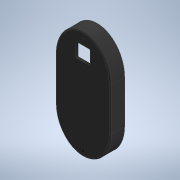
# Autodesk Inventor part: SpectoBoardCap
Saved by Autodesk Inventor 2020 (Build 240168000, 168)
## iProperties
Created: 2019-09-09
Part Number: SpectoBoardCap
Material: ABS Plastic
Document SubType Name: Modeling
Designer: vmiguel
Density: 1.06 g/cm^3
Appearance: Rubber - Black
Author: vmiguel
Autodesk Inventor part; units mm, degrees
ref_plane "YZ Plane" through (0, 0, 0) normal (1, 0, 0) x (0, 1, 0)
ref_plane "XZ Plane" through (0, 0, 0) normal (0, 1, 0) x (-1, 0, 0)
ref_plane "XY Plane" through (0, 0, 0) normal (0, 0, 1) x (1, 0, 0)
sketch "Sketch1" plane through (0, 0, 0) normal (0, 0, 1) x (1, 0, 0)
  ellipse E0 centre (-4, 84.6438) end of major axis (-4, 88.2209) minor radius 3 projected
  ellipse E1 centre (-4, 120.4147) end of major axis (-4, 123.9918) minor radius 3 projected
  line L0 (-23, 113.3579) -> (-23, 147.839) projected
  line L1 (-23, 113.3579) -> (-15.5, 113.3579) projected
  line L2 (-15.5, 113.3579) -> (-15.5, 67.3579) projected
  line L3 (-15.5, 67.3579) -> (-23, 67.3579) projected
  line L4 (-23, 57.2194) -> (-23, 67.3579) projected
  ellipse E2 centre (-23, 84.6438) end of major axis (-23, 57.2194) minor radius 23 (-23, 57.2194) -> (0, 84.6438) ccw projected
  line L5 (0, 120.4147) -> (0, 84.6438) projected
  ellipse E3 centre (-23, 120.4147) end of major axis (-23, 147.839) minor radius 23 (0, 120.4147) -> (-23, 147.839) ccw projected
  ellipse E4 centre (-42, 84.6438) end of major axis (-42, 88.2209) minor radius 3 projected
  ellipse E5 centre (-42, 120.4147) end of major axis (-42, 123.9918) minor radius 3 projected
  line L6 (-23, 113.3579) -> (-23, 147.839) projected
  ellipse E6 centre (-23, 120.4147) end of major axis (-23, 147.839) minor radius 23 (-23, 147.839) -> (-46, 120.4147) ccw projected
  line L7 (-46, 84.6438) -> (-46, 120.4147) projected
  ellipse E7 centre (-23, 84.6438) end of major axis (-23, 57.2194) minor radius 23 (-46, 84.6438) -> (-23, 57.2194) ccw projected
  line L8 (-23, 57.2194) -> (-23, 67.3579) projected
  line L9 (-23, 67.3579) -> (-30.5, 67.3579) projected
  line L10 (-30.5, 67.3579) -> (-30.5, 113.3579) projected
  line L11 (-30.5, 113.3579) -> (-23, 113.3579) projected
  point P0 (0, 0)
  constraints: 8 other
extrude "Extrusion1" add sketch "Sketch1" along normal blind 10 contours E0 | E1 | L11 L10 L9 L4 E7 L7 E6 L0 | L0 E3 L5 E2 L4 L3 L2 L1 | L1 L2 L3 L9 L10 L11 | E4 | E5
sketch "Sketch2" plane through (0, 0, 10) normal (0, 0, 1) x (1, 0, 0)
  ellipse E0 centre (-23, 120.4147) end of major axis (-23, 147.839) minor radius 23 (0, 120.4147) -> (-46, 120.4147) ccw projected
  line L0 (-46, 120.4147) -> (-46, 84.6438) projected
  ellipse E1 centre (-23, 84.6438) end of major axis (-23, 57.2194) minor radius 23 (-46, 84.6438) -> (0, 84.6438) ccw projected
  line L1 (0, 84.6438) -> (0, 120.4147) projected
  line L2 (-3, 120.4147) -> (-3, 84.6438)
  line L3 (-43, 84.6438) -> (-43, 120.4147)
  spline S0 degree 5 poles (-43, 120.4147) (-43, 120.9732) (-42.9869, 121.5316) (-42.9606, 122.0897) (-42.7234, 125.4467) (-42.0085, 128.759) (-41.0798, 131.4357) (-38.6811, 136.2169) (-35.0827, 140.1553) (-33.1335, 141.7599) (-28.9285, 144.1751) (-24.1703, 145.0431) (-21.8297, 145.0431) (-17.0715, 144.1751) (-12.8665, 141.7599) (-10.9173, 140.1553) (-7.3189, 136.2169) (-4.9202, 131.4357) (-3.9915, 128.759) (-3.2766, 125.4467) (-3.0394, 122.0897) (-3.0131, 121.5316) (-3, 120.9732) (-3, 120.4147) knots 0 0 0 0 0 0 0.039929 0.039929 0.039929 0.240547 0.240547 0.240547 0.418246 0.418246 0.418246 0.581754 0.581754 0.581754 0.759453 0.759453 0.759453 0.960071 0.960071 0.960071 1 1 1 1 1 1
  spline S1 degree 5 poles (-3, 84.6438) (-3, 84.0853) (-3.0131, 83.5268) (-3.0394, 82.9688) (-3.2766, 79.6117) (-3.9915, 76.2995) (-4.9202, 73.6227) (-7.3189, 68.8416) (-10.9173, 64.9031) (-12.8665, 63.2985) (-17.0715, 60.8834) (-21.8297, 60.0154) (-24.1703, 60.0154) (-28.9285, 60.8834) (-33.1335, 63.2985) (-35.0827, 64.9031) (-38.6811, 68.8416) (-41.0798, 73.6227) (-42.0085, 76.2995) (-42.7234, 79.6117) (-42.9606, 82.9688) (-42.9869, 83.5268) (-43, 84.0853) (-43, 84.6438) knots 0 0 0 0 0 0 0.039929 0.039929 0.039929 0.240547 0.240547 0.240547 0.418246 0.418246 0.418246 0.581754 0.581754 0.581754 0.759453 0.759453 0.759453 0.960071 0.960071 0.960071 1 1 1 1 1 1
  point P0 (0, 0)
  dimension "d2" = 3
  constraints: 4 end point, 3 parallel, 2 horizontal alignment, 6 other
  measures "d2" distance between parallel lines of L1 L2
extrude "Extrusion2" cut sketch "Sketch2" against normal blind 10 contours L2 S1 L3 S0
sketch "Sketch3" plane through (0, 0, 10) normal (0, 0, 1) x (1, 0, 0)
  line L0 (-43, 84.6438) -> (-43, 120.4147) projected
  line L1 (-3, 120.4147) -> (-3, 84.6438) projected
  ellipse E0 centre (-23, 120.4147) end of major axis (-23, 147.839) minor radius 23 (0, 120.4147) -> (-46, 120.4147) ccw projected
  line L2 (-46, 120.4147) -> (-46, 84.6438) projected
  ellipse E1 centre (-23, 84.6438) end of major axis (-23, 57.2194) minor radius 23 (-46, 84.6438) -> (0, 84.6438) ccw projected
  line L3 (0, 84.6438) -> (0, 120.4147) projected
  point P0 (0, 0)
  constraints: 2 horizontal alignment, 2 other
extrude "Extrusion3" add sketch "Sketch3" along normal blind 2
sketch "Sketch4" plane through (0, 0, 0) normal (0, 0, -1) x (-1, 0, 0)
  circle A0 centre (23, 143.839) radius 4
  circle A1 centre (23, 61.2194) radius 4
  ellipse E0 centre (23, 120.4147) end of major axis (23, 147.839) minor radius 23 (46, 120.4147) -> (0, 120.4147) ccw projected
  ellipse E1 centre (23, 84.6438) end of major axis (23, 57.2194) minor radius 23 (0, 84.6438) -> (46, 84.6438) ccw projected
  point P0 (0, 0)
  dimension "d7" = 8
  dimension "d8" = 8
  constraints: 2 centre point, 2 vertical alignment, 4 other
  measures "d7" diameter of A0
  measures "d8" diameter of A1
extrude "Extrusion4" add sketch "Sketch4" against normal blind 10
fillet "Fillet1" radius 2 4 edges at (-19.0329, 60.7071, 5) (-26.9671, 60.7071, 5) (-26.9671, 144.3514, 5) (-19.0329, 144.3514, 5)
sketch "Sketch5" plane through (0, 0, 0) normal (0, 0, -1) x (-1, 0, 0)
  arc A0 (19.26, 142.4204) -> (26.74, 142.4204) centre (23, 143.839) ccw projected
  arc A1 (26.74, 62.6381) -> (19.26, 62.6381) centre (23, 61.2194) ccw projected
  point P0 (0, 0)
  constraints: 2 coincident
hole "Hole1" at (-23, 143.839, 0) at (-23, 61.2194, 0) direction (0, 0, 1) diameter 3 end through all
sketch "Sketch6" plane through (0, 0, 12) normal (0, 0, 1) x (1, 0, 0)
  line L0 (-28.5, 137.839) -> (-17.5, 137.839)
  line L1 (-17, 137.339) -> (-17, 126.339)
  line L2 (-17.5, 125.839) -> (-28.5, 125.839)
  line L3 (-29, 126.339) -> (-29, 137.339)
  line L4 (-29, 137.839) -> (-17, 125.839) construction
  line L5 (-17, 137.839) -> (-29, 125.839) construction
  arc A0 (-28.5, 137.839) -> (-29, 137.339) centre (-28.5, 137.339) ccw
  arc A1 (-29, 126.339) -> (-28.5, 125.839) centre (-28.5, 126.339) ccw
  arc A2 (-17.5, 125.839) -> (-17, 126.339) centre (-17.5, 126.339) ccw
  arc A3 (-17, 137.339) -> (-17.5, 137.839) centre (-17.5, 137.339) ccw
  circle A4 centre (-23, 143.839) radius 1.5 projected
  point P0 (0, 0)
  point P1 (-23, 131.839)
  point P2 (-23, 131.839)
  dimension "d19" = 12
  dimension "d20" = 12
  dimension "d21" = 0.5
  dimension "d22" = 6
  constraints: 12 end point, 8 point on circle, 8 point on line, 8 tangent, 4 centre point, 3 equal radius, 3 midpoint, 2 parallel, 1 horizontal, 1 perpendicular, 1 vertical alignment
  measures "d19" distance of L4.end L5.end
  measures "d20" distance of L5.start L4.end
  measures "d21" radius of A0
  measures "d22" distance from line of L0 A4.centre
extrude "Extrusion5" cut sketch "Sketch6" against normal blind 10 contours L0 A3 L1 A2 L2 A1 L3 A0
fillet "Fillet2" radius 1 4 edges at (-46, 102.5292, 12) (-23, 57.2194, 12) (0, 102.5292, 12) (-23, 147.839, 12)
body "Solid1"
